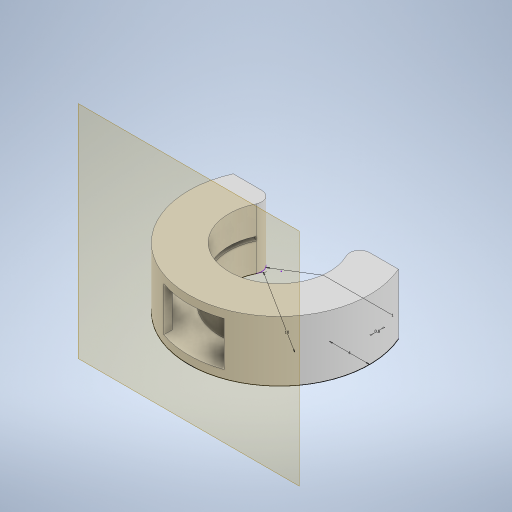
# Autodesk Inventor part: ir다이오드꼽는부분
Saved by Autodesk Inventor 2023 (Build 270158000, 158)
## iProperties
Created: 2023-04-25
Part Number: ir다이오드꼽는부분
Material: 일반
Document SubType Name: Modeling
Designer: rlatk
Density: 1 g/cm^3
Appearance: 기본값
Author: rlatk
Autodesk Inventor part; units mm, degrees
ref_plane "YZ Plane" through (0, 0, 0) normal (1, 0, 0) x (0, 1, 0)
ref_plane "XZ Plane" through (0, 0, 0) normal (0, 1, 0) x (-1, 0, 0)
ref_plane "XY Plane" through (0, 0, 0) normal (0, 0, 1) x (1, 0, 0)
sketch "스케치1" plane through (0, 0, 0) normal (0, 1, 0) x (-1, 0, 0)
  arc A0 (4.4849, -2.2103) -> (-4.4849, -2.2103) centre (0, 0) ccw
  arc A1 (8.2256, -3.6523) -> (-8.2256, -3.6523) centre (0, 0) ccw
  line L0 (8.2256, -3.6523) -> (5.3819, -3.6523)
  line L1 (-5.3819, -3.6523) -> (-8.2256, -3.6523)
  arc A2 (4.4849, -2.2103) -> (5.3819, -3.6523) centre (5.3819, -2.6523) ccw
  arc A3 (-5.3819, -3.6523) -> (-4.4849, -2.2103) centre (-5.3819, -2.6523) ccw
  arc A4 (7.6879, -2.8523) -> (-7.6879, -2.8523) centre (0, 0) ccw
  line L2 (7.6879, -2.8523) -> (5.3819, -2.8523)
  arc A5 (5.2025, -2.5639) -> (5.3819, -2.8523) centre (5.3819, -2.6523) ccw
  arc A6 (5.2025, -2.5639) -> (-5.2025, -2.5639) centre (0, 0) ccw
  arc A7 (-5.3819, -2.8523) -> (-5.2025, -2.5639) centre (-5.3819, -2.6523) ccw
  line L3 (-5.3819, -2.8523) -> (-7.6879, -2.8523)
  line L4 (-5.2025, -2.5639) -> (-4.4849, -2.2103)
  line L5 (5.2025, -2.5639) -> (4.4849, -2.2103)
  point P0 (-3.4148, -3.6523)
  point P1 (3.4148, -3.6523)
  dimension "d0" = 10
  dimension "d1" = 4
  dimension "d2" = 1
  dimension "d5" = 0.8
  constraints: 18 point on circle, 12 end point, 8 centre point, 4 tangent, 2 horizontal, 2 point on line, 1 coincident, 1 equal radius, 5 other
  measures "d0" diameter of A0
  measures "d1" radial gap between concentric circles of A0 A1
  measures "d2" radius of A2
  measures "d5" distance between parallel lines of L1 L3
extrude "돌출1" add sketch "스케치1" along normal blind 6
extrude "돌출2" cut sketch "스케치1" along normal blind 5.2 contours A6 A7 L3 A4 L2 A5
extrude "돌출3" add sketch "스케치1" along normal blind 0.8 contours A6 A7 L3 A4 L2 A5
sketch "스케치2" plane through (0, 0, 0) normal (0, -1, 0) x (1, 0, 0)
  point P0 (0, 0)
extrude "돌출4" cut sketch "스케치1" along normal blind 3.2 contours A0 L4 A6 L5
extrude "돌출5" add sketch "스케치1" along normal blind 2.8 contours A0 L4 A6 L5
ref_plane "작업 평면1" through (0, 6, 9) normal (0, 0, 1) x (1, 0, 0)
sketch "스케치3" plane through (0, 6, 9) normal (0, 0, 1) x (1, 0, 0)
  line L0 (8.2, -0.8) -> (-8.2, -0.8) projected
  line L1 (-8.2, -5.2) -> (8.2, -5.2) projected
  line L2 (-8.2, -5.2) -> (-8.2, -0.8) projected
  line L3 (8.2, -5.2) -> (8.2, -0.8) projected
  line L4 (0, -5.2) -> (-3, -5.2)
  line L5 (-3, -5.2) -> (-3, -0.8)
  line L6 (-3, -0.8) -> (0, -0.8)
  line L7 (-8.2, -0.8) -> (8.2, -0.8)
  line L8 (8.2, -5.2) -> (-8.2, -5.2)
  line L9 (3, -5.2) -> (3, -0.8)
  point P0 (0, -6)
  point P1 (-7.6879, -0.8)
  point P2 (7.6879, -0.8)
  point P3 (7.6879, -5.2)
  point P4 (-7.6879, -5.2)
  dimension "d14" = 3
  constraints: 12 end point, 4 point on line, 2 midpoint, 1 perpendicular
  measures "d14" distance of L4.start L4.end
extrude "돌출6" cut sketch "스케치3" against normal blind 3.2 contours L9 L1 L5 L0
